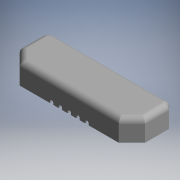
# Autodesk Inventor part: Box
Saved by Autodesk Inventor 2018.3 (Build 223284000, 284)
## iProperties
Part Number: Box
Material: Generic
Document SubType Name: Modeling
Designer: Gregor Gombač
Mass: 2.57152 g
Surface Area: 42.7836 cm^2
Volume: 2.57152 cm^3
Density: 1 g/cm^3
Appearance: Generic
Author: Gregor Gombač
Autodesk Inventor part; units mm, degrees
ref_plane "YZ Plane" through (0, 0, 0) normal (1, 0, 0) x (0, 1, 0)
ref_plane "XZ Plane" through (0, 0, 0) normal (0, 1, 0) x (-1, 0, 0)
ref_plane "XY Plane" through (0, 0, 0) normal (0, 0, 1) x (1, 0, 0)
sketch "Sketch1" plane through (0, 0, 0) normal (0, 1, 0) x (-1, 0, 0)
  line L0 (22.125, 8.625) -> (-22.125, 8.625)
  line L1 (-22.125, 8.625) -> (-27.625, 3.125)
  line L2 (-27.625, 3.125) -> (-27.625, -7.125)
  line L3 (-27.625, -7.125) -> (-26.125, -8.625)
  line L4 (-26.125, -8.625) -> (26.125, -8.625)
  line L5 (26.125, -8.625) -> (27.625, -7.125)
  line L6 (27.625, -7.125) -> (27.625, 3.125)
  line L7 (27.625, 3.125) -> (22.125, 8.625)
  line L8 (27.625, 3.125) -> (27.625, 8.625) construction
  line L9 (27.625, 8.625) -> (22.125, 8.625) construction
  line L10 (-26.125, -8.625) -> (-27.625, -8.625) construction
  line L11 (-27.625, -8.625) -> (-27.625, -7.125) construction
  line L12 (-27.625, 3.125) -> (-27.625, 8.625) construction
  line L13 (-27.625, 8.625) -> (-22.125, 8.625) construction
  line L14 (27.625, -7.125) -> (27.625, -8.625) construction
  line L15 (27.625, -8.625) -> (26.125, -8.625) construction
  line L16 (27.625, 8.625) -> (-27.625, -8.625) construction
  line L17 (27.625, -8.625) -> (-27.625, 8.625) construction
  line L18 (26.4357, -9.375) -> (-26.4357, -9.375)
  line L19 (-26.4357, -9.375) -> (-28.375, -7.4357)
  line L20 (-28.375, -7.4357) -> (-28.375, 3.4357)
  line L21 (-28.375, 3.4357) -> (-22.4357, 9.375)
  line L22 (-22.4357, 9.375) -> (22.4357, 9.375)
  line L23 (22.4357, 9.375) -> (28.375, 3.4357)
  line L24 (28.375, 3.4357) -> (28.375, -7.4357)
  line L25 (28.375, -7.4357) -> (26.4357, -9.375)
  point P0 (0, 0)
  point P1 (0, 0)
  dimension "d1" = 135
  dimension "d2" = 52.25
  dimension "d3" = 44.25
  dimension "d4" = 10.25
  dimension "d5" = 17.25
  dimension "d7" = 0.75
  constraints: 52 end point, 7 collinear, 7 parallel, 2 equal length, 2 horizontal, 2 perpendicular, 1 coincident, 1 midpoint, 1 vertical, 7 other
  measures "d1" angle of L3 L4
  measures "d2" distance of L3.end L4.end
  measures "d3" distance of L0.start L0.end
  measures "d4" distance of L5.end L6.end
  measures "d5" distance between parallel lines of L0 L4
  measures "d7" distance between parallel lines of L4 L18
extrude "Extrusion1" add sketch "Sketch1" along normal blind 5 contours L7 L6 L5 L4 L3 L2 L1 L0 | L18 L19 L20 L21 L22 L23 L24 L25
fillet "Fillet1" radius 2.5 8 edges at (0, 5, -9.375) (-27.4053, 5, -8.4053) (-28.375, 5, -2) (-25.4053, 5, 6.4053) (0, 5, 9.375) (25.4053, 5, 6.4053) (28.375, 5, -2) (27.4053, 5, -8.4053)
shell "Shell1" thickness 1.5 removed faces 1 at (7.4786, 0, -3.125)
extrude "Extrusion2" add sketch "Sketch1" against normal blind 4.6
sketch "Sketch2" plane through (26.4357, 2.5, 9.375) normal (0, 0, -1) x (-1, 0, 0)
  line L0 (52.8713, -7.1) -> (0, -7.1) construction
  line L1 (35.1857, -7.1) -> (35.1857, -6.35)
  arc A0 (35.1857, -6.35) -> (33.6857, -6.35) centre (34.4357, -6.35) ccw
  line L2 (33.6857, -6.35) -> (33.6857, -7.1)
  line L3 (31.1857, -7.1) -> (31.1857, -6.35)
  arc A1 (31.1857, -6.35) -> (29.6857, -6.35) centre (30.4357, -6.35) ccw
  line L4 (29.6857, -6.35) -> (29.6857, -7.1)
  line L5 (27.1857, -7.1) -> (27.1857, -6.35)
  arc A2 (27.1857, -6.35) -> (25.6857, -6.35) centre (26.4357, -6.35) ccw
  line L6 (25.6857, -6.35) -> (25.6857, -7.1)
  line L7 (23.1857, -7.1) -> (23.1857, -6.35)
  arc A3 (23.1857, -6.35) -> (21.6857, -6.35) centre (22.4357, -6.35) ccw
  line L8 (21.6857, -6.35) -> (21.6857, -7.1)
  line L9 (19.1857, -7.1) -> (19.1857, -6.35)
  arc A4 (19.1857, -6.35) -> (17.6857, -6.35) centre (18.4357, -6.35) ccw
  line L10 (17.6857, -6.35) -> (17.6857, -7.1)
  line L11 (35.1857, -7.1) -> (33.6857, -7.1)
  line L12 (31.1857, -7.1) -> (29.6857, -7.1)
  line L13 (27.1857, -7.1) -> (25.6857, -7.1)
  line L14 (23.1857, -7.1) -> (21.6857, -7.1)
  line L15 (19.1857, -7.1) -> (17.6857, -7.1)
  point P0 (26.4357, -2.5)
  dimension "d14" = 1.5
  dimension "d15" = 0.75
  dimension "d18" = 4
  constraints: 30 end point, 10 point on circle, 5 centre point, 5 collinear, 2 point on line, 2 tangent, 1 horizontal, 1 perpendicular, 1 vertical, 1 vertical alignment, 32 other
  measures "d14" distance between parallel lines of L2 L1
  measures "d15" distance of L1.start L1.end
  measures "d18" distance of L1.start L3.start
extrude "Extrusion3" cut sketch "Sketch2" along normal up to next
equation "\"d15\" = 0.5 * d14"
body "Solid1"
